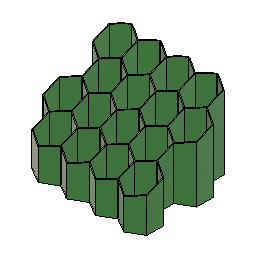
hexagon-05 (Autodesk Fusion 360 design; units mm, degrees)
Autodesk Fusion 360 part; units mm, degrees
note: some values were not read from the file. Set by a fixed rule: which sketch regions a step uses.
sketch "Sketch1" plane through (0, 0, 0) normal (0, 1, 0) x (1, 0, 0)
  line L0 (15.0321, 8.6045) -> (0.0644, 17.3204)
  line L1 (0.0644, 17.3204) -> (-14.9677, 8.7159)
  line L2 (-14.9677, 8.7159) -> (-15.0321, -8.6045)
  line L3 (-15.0321, -8.6045) -> (-0.0644, -17.3204)
  line L4 (-0.0644, -17.3204) -> (14.9677, -8.7159)
  line L5 (14.9677, -8.7159) -> (15.0321, 8.6045)
  line L6 (14.9677, -8.7159) -> (-0.0644, -17.3204)
  line L7 (-0.0644, -17.3204) -> (-0.1287, -34.6408)
  line L8 (-0.1287, -34.6408) -> (14.839, -43.3567)
  line L9 (14.839, -43.3567) -> (29.8711, -34.7523)
  line L10 (29.8711, -34.7523) -> (29.9354, -17.4319)
  line L11 (29.9354, -17.4319) -> (14.9677, -8.7159)
  line L12 (14.839, -43.3567) -> (-0.1287, -34.6408)
  line L13 (-0.1287, -34.6408) -> (-15.1608, -43.2452)
  line L14 (-15.1608, -43.2452) -> (-15.2252, -60.5656)
  line L15 (-15.2252, -60.5656) -> (-0.2575, -69.2816)
  line L16 (-0.2575, -69.2816) -> (14.7746, -60.6771)
  line L17 (14.7746, -60.6771) -> (14.839, -43.3567)
  line L18 (14.6, 8.4293) -> (0, 16.8586)
  line L19 (0, 16.8586) -> (-14.6, 8.4293)
  line L20 (-14.6, 8.4293) -> (-14.6, -8.4293)
  line L21 (-14.6, -8.4293) -> (0, -16.8586)
  line L22 (0, -16.8586) -> (14.6, -8.4293)
  line L23 (14.6, -8.4293) -> (14.6, 8.4293)
  line L24 (29.5033, -17.607) -> (14.9033, -9.1777)
  line L25 (14.9033, -9.1777) -> (0.3033, -17.607)
  line L26 (0.3033, -17.607) -> (0.3033, -34.4656)
  line L27 (0.3033, -34.4656) -> (14.9033, -42.895)
  line L28 (14.9033, -42.895) -> (29.5033, -34.4656)
  line L29 (29.5033, -34.4656) -> (29.5033, -17.607)
  line L30 (14.4069, -43.5319) -> (-0.1931, -35.1025)
  line L31 (-0.1931, -35.1025) -> (-14.7931, -43.5319)
  line L32 (-14.7931, -43.5319) -> (-14.7931, -60.3905)
  line L33 (-14.7931, -60.3905) -> (-0.1931, -68.8198)
  line L34 (-0.1931, -68.8198) -> (14.4069, -60.3905)
  line L35 (14.4069, -60.3905) -> (14.4069, -43.5319)
  line L36 (14.7746, -60.6771) -> (-0.2575, -69.2816)
  line L37 (-0.2575, -69.2816) -> (-0.3218, -86.6019)
  line L38 (-0.3218, -86.6019) -> (14.6459, -95.3179)
  line L39 (14.6459, -95.3179) -> (29.678, -86.7134)
  line L40 (29.678, -86.7134) -> (29.7423, -69.393)
  line L41 (29.7423, -69.393) -> (14.7746, -60.6771)
  line L42 (29.3103, -69.5682) -> (14.7103, -61.1389)
  line L43 (14.7103, -61.1389) -> (0.1103, -69.5682)
  line L44 (0.1103, -69.5682) -> (0.1103, -86.4268)
  line L45 (0.1103, -86.4268) -> (14.7103, -94.8561)
  line L46 (14.7103, -94.8561) -> (29.3103, -86.4268)
  line L47 (29.3103, -86.4268) -> (29.3103, -69.5682)
  line L48 (44.7746, -60.6771) -> (29.7425, -69.2816)
  line L49 (44.9677, -8.7159) -> (45.0321, 8.6045)
  line L50 (44.9033, -9.1777) -> (30.3033, -17.607)
  line L51 (29.9356, -17.3204) -> (44.9677, -8.7159)
  line L52 (15.4, 8.4293) -> (15.4, -8.4293)
  line L53 (14.7748, -60.5656) -> (29.7425, -69.2816)
  line L54 (30, -16.8586) -> (44.6, -8.4293)
  line L55 (29.7425, -69.2816) -> (29.6782, -86.6019)
  line L56 (44.7103, -61.1389) -> (30.1103, -69.5682)
  line L57 (29.8069, -68.8198) -> (44.4069, -60.3905)
  line L58 (45.0321, 8.6045) -> (30.0644, 17.3204)
  line L59 (15.0323, 8.7159) -> (14.9679, -8.6045)
  line L60 (30.1103, -69.5682) -> (30.1103, -86.4268)
  line L61 (30.3033, -17.607) -> (30.3033, -34.4656)
  line L62 (29.8713, -34.6408) -> (14.8392, -43.2452)
  line L63 (15.4, -8.4293) -> (30, -16.8586)
  line L64 (30, 16.8586) -> (15.4, 8.4293)
  line L65 (29.8069, -35.1025) -> (15.2069, -43.5319)
  line L66 (44.839, -43.3567) -> (29.8713, -34.6408)
  line L67 (30.0644, 17.3204) -> (15.0323, 8.7159)
  line L68 (44.4069, -43.5319) -> (29.8069, -35.1025)
  line L69 (29.9356, -17.3204) -> (29.8713, -34.6408)
  line L70 (44.6, -8.4293) -> (44.6, 8.4293)
  line L71 (30.3033, -34.4656) -> (44.9033, -42.895)
  line L72 (44.9677, -8.7159) -> (29.9356, -17.3204)
  line L73 (44.6, 8.4293) -> (30, 16.8586)
  line L74 (59.3103, -69.5682) -> (44.7103, -61.1389)
  line L75 (59.9354, -17.4319) -> (44.9677, -8.7159)
  line L76 (59.7423, -69.393) -> (44.7746, -60.6771)
  line L77 (44.9033, -42.895) -> (59.5033, -34.4656)
  line L78 (59.678, -86.7134) -> (59.7423, -69.393)
  line L79 (59.5033, -17.607) -> (44.9033, -9.1777)
  line L80 (44.6459, -95.3179) -> (59.678, -86.7134)
  line L81 (44.839, -43.3567) -> (59.8711, -34.7523)
  line L82 (59.8711, -34.7523) -> (59.9354, -17.4319)
  line L83 (59.5033, -34.4656) -> (59.5033, -17.607)
  line L84 (15.2069, -60.3905) -> (29.8069, -68.8198)
  line L85 (44.4069, -60.3905) -> (44.4069, -43.5319)
  line L86 (29.6782, -86.6019) -> (44.6459, -95.3179)
  line L87 (30.1103, -86.4268) -> (44.7103, -94.8561)
  line L88 (14.9679, -8.6045) -> (29.9356, -17.3204)
  line L89 (29.7425, -69.2816) -> (44.7746, -60.6771)
  line L90 (29.8713, -34.6408) -> (44.839, -43.3567)
  line L91 (59.3103, -86.4268) -> (59.3103, -69.5682)
  line L92 (44.7103, -94.8561) -> (59.3103, -86.4268)
  line L93 (44.7746, -60.6771) -> (44.839, -43.3567)
  line L94 (14.8392, -43.2452) -> (14.7748, -60.5656)
  line L95 (15.2069, -43.5319) -> (15.2069, -60.3905)
  line L96 (74.7746, -60.6771) -> (59.7425, -69.2816)
  line L97 (74.9677, -8.7159) -> (75.0321, 8.6045)
  line L98 (74.9033, -9.1777) -> (60.3033, -17.607)
  line L99 (59.9356, -17.3204) -> (74.9677, -8.7159)
  line L100 (45.4, 8.4293) -> (45.4, -8.4293)
  line L101 (44.7748, -60.5656) -> (59.7425, -69.2816)
  line L102 (60, -16.8586) -> (74.6, -8.4293)
  line L103 (59.7425, -69.2816) -> (59.6782, -86.6019)
  line L104 (74.7103, -61.1389) -> (60.1103, -69.5682)
  line L105 (59.8069, -68.8198) -> (74.4069, -60.3905)
  line L106 (75.0321, 8.6045) -> (60.0644, 17.3204)
  line L107 (45.0323, 8.7159) -> (44.9679, -8.6045)
  line L108 (60.1103, -69.5682) -> (60.1103, -86.4268)
  line L109 (60.3033, -17.607) -> (60.3033, -34.4656)
  line L110 (59.8713, -34.6408) -> (44.8392, -43.2452)
  line L111 (45.4, -8.4293) -> (60, -16.8586)
  line L112 (60, 16.8586) -> (45.4, 8.4293)
  line L113 (59.8069, -35.1025) -> (45.2069, -43.5319)
  line L114 (74.839, -43.3567) -> (59.8713, -34.6408)
  line L115 (60.0644, 17.3204) -> (45.0323, 8.7159)
  line L116 (74.4069, -43.5319) -> (59.8069, -35.1025)
  line L117 (59.9356, -17.3204) -> (59.8713, -34.6408)
  line L118 (74.6, -8.4293) -> (74.6, 8.4293)
  line L119 (60.3033, -34.4656) -> (74.9033, -42.895)
  line L120 (74.9677, -8.7159) -> (59.9356, -17.3204)
  line L121 (74.6, 8.4293) -> (60, 16.8586)
  line L122 (89.3103, -69.5682) -> (74.7103, -61.1389)
  line L123 (89.9354, -17.4319) -> (74.9677, -8.7159)
  line L124 (89.7423, -69.393) -> (74.7746, -60.6771)
  line L125 (74.9033, -42.895) -> (89.5033, -34.4656)
  line L126 (89.678, -86.7134) -> (89.7423, -69.393)
  line L127 (89.5033, -17.607) -> (74.9033, -9.1777)
  line L128 (74.6459, -95.3179) -> (89.678, -86.7134)
  line L129 (74.839, -43.3567) -> (89.8711, -34.7523)
  line L130 (89.8711, -34.7523) -> (89.9354, -17.4319)
  line L131 (89.5033, -34.4656) -> (89.5033, -17.607)
  line L132 (45.2069, -60.3905) -> (59.8069, -68.8198)
  line L133 (74.4069, -60.3905) -> (74.4069, -43.5319)
  line L134 (59.6782, -86.6019) -> (74.6459, -95.3179)
  line L135 (60.1103, -86.4268) -> (74.7103, -94.8561)
  line L136 (44.9679, -8.6045) -> (59.9356, -17.3204)
  line L137 (59.7425, -69.2816) -> (74.7746, -60.6771)
  line L138 (59.8713, -34.6408) -> (74.839, -43.3567)
  line L139 (89.3103, -86.4268) -> (89.3103, -69.5682)
  line L140 (74.7103, -94.8561) -> (89.3103, -86.4268)
  line L141 (74.7746, -60.6771) -> (74.839, -43.3567)
  line L142 (44.8392, -43.2452) -> (44.7748, -60.5656)
  line L143 (45.2069, -43.5319) -> (45.2069, -60.3905)
  line L144 (104.7746, -60.6771) -> (89.7425, -69.2816)
  line L145 (104.9677, -8.7159) -> (105.0321, 8.6045)
  line L146 (104.9033, -9.1777) -> (90.3033, -17.607)
  line L147 (89.9356, -17.3204) -> (104.9677, -8.7159)
  line L148 (75.4, 8.4293) -> (75.4, -8.4293)
  line L149 (74.7748, -60.5656) -> (89.7425, -69.2816)
  line L150 (90, -16.8586) -> (104.6, -8.4293)
  line L151 (89.7425, -69.2816) -> (89.6782, -86.6019)
  line L152 (104.7103, -61.1389) -> (90.1103, -69.5682)
  line L153 (89.8069, -68.8198) -> (104.4069, -60.3905)
  line L154 (105.0321, 8.6045) -> (90.0644, 17.3204)
  line L155 (75.0323, 8.7159) -> (74.9679, -8.6045)
  line L156 (90.1103, -69.5682) -> (90.1103, -86.4268)
  line L157 (90.3033, -17.607) -> (90.3033, -34.4656)
  line L158 (89.8713, -34.6408) -> (74.8392, -43.2452)
  line L159 (75.4, -8.4293) -> (90, -16.8586)
  line L160 (90, 16.8586) -> (75.4, 8.4293)
  line L161 (89.8069, -35.1025) -> (75.2069, -43.5319)
  line L162 (104.839, -43.3567) -> (89.8713, -34.6408)
  line L163 (90.0644, 17.3204) -> (75.0323, 8.7159)
  line L164 (104.4069, -43.5319) -> (89.8069, -35.1025)
  line L165 (89.9356, -17.3204) -> (89.8713, -34.6408)
  line L166 (104.6, -8.4293) -> (104.6, 8.4293)
  line L167 (90.3033, -34.4656) -> (104.9033, -42.895)
  line L168 (104.9677, -8.7159) -> (89.9356, -17.3204)
  line L169 (104.6, 8.4293) -> (90, 16.8586)
  line L170 (119.3103, -69.5682) -> (104.7103, -61.1389)
  line L171 (119.9354, -17.4319) -> (104.9677, -8.7159)
  line L172 (119.7423, -69.393) -> (104.7746, -60.6771)
  line L173 (104.9033, -42.895) -> (119.5033, -34.4656)
  line L174 (119.678, -86.7134) -> (119.7423, -69.393)
  line L175 (119.5033, -17.607) -> (104.9033, -9.1777)
  line L176 (104.6459, -95.3179) -> (119.678, -86.7134)
  line L177 (104.839, -43.3567) -> (119.8711, -34.7523)
  line L178 (119.8711, -34.7523) -> (119.9354, -17.4319)
  line L179 (119.5033, -34.4656) -> (119.5033, -17.607)
  line L180 (75.2069, -60.3905) -> (89.8069, -68.8198)
  line L181 (104.4069, -60.3905) -> (104.4069, -43.5319)
  line L182 (89.6782, -86.6019) -> (104.6459, -95.3179)
  line L183 (90.1103, -86.4268) -> (104.7103, -94.8561)
  line L184 (74.9679, -8.6045) -> (89.9356, -17.3204)
  line L185 (89.7425, -69.2816) -> (104.7746, -60.6771)
  line L186 (89.8713, -34.6408) -> (104.839, -43.3567)
  line L187 (119.3103, -86.4268) -> (119.3103, -69.5682)
  line L188 (104.7103, -94.8561) -> (119.3103, -86.4268)
  line L189 (104.7746, -60.6771) -> (104.839, -43.3567)
  line L190 (74.8392, -43.2452) -> (74.7748, -60.5656)
  line L191 (75.2069, -43.5319) -> (75.2069, -60.3905)
  point P0 (14.9033, -26.0363)
  point P1 (-0.1931, -51.9612)
  point P2 (14.9033, -26.0363)
  point P3 (-0.1931, -51.9612)
  point P4 (14.7103, -77.9975)
  point P5 (14.7103, -77.9975)
  point P6 (44.9033, -26.0363)
  point P7 (29.8069, -51.9612)
  point P8 (44.9033, -26.0363)
  point P9 (30, 0)
  point P10 (30, 0)
  point P11 (29.8069, -51.9612)
  point P12 (44.7103, -77.9975)
  point P13 (30, 0)
  point P14 (44.7103, -77.9975)
  point P15 (74.9033, -26.0363)
  point P16 (59.8069, -51.9612)
  point P17 (74.9033, -26.0363)
  point P18 (60, 0)
  point P19 (60, 0)
  point P20 (59.8069, -51.9612)
  point P21 (74.7103, -77.9975)
  point P22 (60, 0)
  point P23 (74.7103, -77.9975)
  point P24 (104.9033, -26.0363)
  point P25 (89.8069, -51.9612)
  point P26 (104.9033, -26.0363)
  point P27 (90, 0)
  point P28 (90, 0)
  point P29 (89.8069, -51.9612)
  point P30 (104.7103, -77.9975)
  point P31 (90, 0)
  point P32 (104.7103, -77.9975)
  dimension "d29" = 15
  dimension "d30" = 14.6
  dimension "d31" = 14.6
  dimension "d32" = 14.6
  dimension "d33" = 14.6
  dimension "d36" = 90
  dimension "d37" = 0
  constraint coincident P2 P0
  constraint coincident P3 P1
  constraint coincident P5 P4
  measures "d29" distance of origin L5
  measures "d30" distance of origin L23
  measures "d31" distance of P2 L29
  measures "d32" distance of P3 L35
  measures "d33" distance of P5 L47
extrude "Extrude2" add sketch "Sketch1" along normal blind 1 contours L0 L1 L2 L3 L4 L5 L6 L59 | L5 L49 L51 L58 L59 L67 L72 L88 L107 | L5 L11 L69 L88 | L4 L6 L7 L8 L10 L11 L12 L62 L69 L94 | L10 L51 L66 L69 L72 L75 L82 L90 L110 L117 L142 | L49 L75 L117 L136 | L49 L97 L99 L106 L107 L115 L120 L136 L155 | L8 L12 L13 L14 L15 L16 L17 L36 L94 | L9 L10 L17 L48 L53 L66 L89 L90 L93 L94 L142 | L9 L10 L62 L94 | L82 L99 L114 L117 L120 L123 L130 L138 L158 L165 L190 | L81 L82 L110 L142 | L81 L82 L93 L96 L101 L114 L137 L138 L141 L142 L190 | L17 L41 L53 L55 | L76 L93 L101 L103 | L97 L123 L165 L184 | L129 L130 L158 L190 | L129 L130 L141 L144 L149 L162 L185 L186 L189 L190 | L97 L145 L147 L154 L155 L163 L168 L184 | L16 L36 L37 L38 L39 L40 L41 L55 | L40 L48 L55 L76 L78 L80 L86 L89 L103 | L78 L96 L103 L124 L126 L128 L134 L137 L151 | L130 L147 L162 L165 L168 L171 L177 L178 L186 | L124 L141 L149 L151 | L126 L144 L151 L172 L174 L176 L182 L185 | L18 L19 L20 L21 L22 L23 | L24 L25 L26 L27 L28 L29 | L30 L31 L32 L33 L34 L35 | L42 L43 L44 L45 L46 L47 | L50 L61 L71 L77 L79 L83 | L52 L54 L63 L64 L70 L73 | L56 L60 L74 L87 L91 L92 | L57 L65 L68 L84 L85 L95 | L98 L109 L119 L125 L127 L131 | L100 L102 L111 L112 L118 L121 | L104 L108 L122 L135 L139 L140 | L105 L113 L116 L132 L133 L143 | L146 L157 L167 L173 L175 L179 | L148 L150 L159 L160 L166 L169 | L152 L156 L170 L183 L187 L188 | L153 L161 L164 L180 L181 L191 makes body 1
extrude "Extrude3" add sketch "Sketch1" along normal blind 80 bodies 1
sketch "Sketch2" plane through (0, 0, 0) normal (1, 0, 0) x (0, 0, -1)
  line L0 (29.2937, 86.3188) -> (-96.3109, 32.1145)
  line L1 (-96.3109, 32.1145) -> (-96.3109, 86.3188)
  line L2 (-96.3109, 86.3188) -> (29.2937, 86.3188)
  constraint vertical L1
  constraint perpendicular L1 L2
extrude "Extrude4" cut sketch "Sketch2" along normal blind 159 and the other way blind 41 bodies 1
copy_body "Body->Comp1" bodies 1 removing the originals makes body 2 in component "hexagon-05"
move_face "OffsetFaces1" offset 0.4 30 faces at (10.0428, 25.7968, -11.5098) (20.043, 25.8129, -11.5841) (40.0428, 25.7968, -11.5098) (50.043, 25.8129, -11.5841) (70.0428, 25.7968, -11.5098) (80.043, 25.8129, -11.5841) (100.0428, 25.7968, -11.5098) (105.0106, 49.1021, -2.831) (109.957, 45.3568, 11.6212) (119.914, 41.6115, 23.2053) (114.8604, 37.8822, 37.6204) (104.8175, 34.153, 49.1302) (109.7639, 30.4077, 63.5824) (119.7209, 26.6624, 75.1665) (114.6673, 22.9331, 89.5816) (94.6674, 22.9491, 89.5073) (84.6673, 22.9331, 89.5816) (64.6674, 22.9491, 89.5073) (54.6673, 22.9331, 89.5816) (34.6674, 22.9491, 89.5073) (24.6673, 22.9331, 89.5816) (4.6674, 22.9491, 89.5073) (-0.2789, 26.6944, 75.055) (-10.2359, 30.4397, 63.4709) (-15.1823, 34.185, 49.0187) (-5.1394, 37.9143, 37.5089) (-0.0858, 41.6436, 23.0939) (-10.0428, 45.3889, 11.5098) (-14.9892, 49.1342, -2.9425) (-9.957, 25.8129, -11.5841) on bodies 2 in component "hexagon-05"
component "hexagon-05" placed x (1, 0, 0) y (0, 1, 0) z (0, 0, 1) at (0, 0, 0)
equation "size1 = 15 mm"
equation "offset1 = 0.4 mm"
equation "d29 = size1"
equation "d30 = size1 - offset1"
equation "d31 = size1 - offset1"
equation "d32 = size1 - offset1"
equation "d33 = size1 - offset1"
equation "d36 = 6 * size1"
equation "d38 = base"
equation "d40 = height"
equation "height = 80 mm"
equation "base = 1 mm"
equation "d48 = expansion"
equation "expansion = 0.4 mm"
